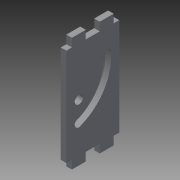
# Autodesk Inventor part: side.plate.cam.rev3
Saved by Autodesk Inventor 2015 SP1 (Build 190203100, 203)
## iProperties
Created: 2016-03-08
Part Number: side.plate.cam.rev3
Material: Generic
Document SubType Name: Modeling
Designer: 200288284
Density: 1 g/cm^3
Appearance: Default
Author: 200288284
Autodesk Inventor part; units mm, degrees
ref_plane "YZ Plane" through (0, 0, 0) normal (1, 0, 0) x (0, 1, 0)
ref_plane "XZ Plane" through (0, 0, 0) normal (0, 1, 0) x (-1, 0, 0)
ref_plane "XY Plane" through (0, 0, 0) normal (0, 0, 1) x (1, 0, 0)
sketch "Sketch1" plane through (0, 0, 0) normal (1, 0, 0) x (0, 1, 0)
  line L0 (8.4448, 10.1682) -> (-26.5552, 10.1682)
  line L1 (-26.5552, 10.1682) -> (-26.5552, 8.1682)
  line L2 (-26.5552, 8.1682) -> (-29.5552, 8.1682)
  line L3 (-29.5552, 8.1682) -> (-29.5552, 3.1682)
  line L4 (-29.5552, 3.1682) -> (-26.5552, 3.1682)
  line L5 (-26.5552, 3.1682) -> (-26.5552, -1.8356)
  line L6 (-26.5552, -1.8356) -> (-29.5552, -1.8356)
  line L7 (-29.5552, -1.8356) -> (-29.5552, -6.8356)
  line L8 (-29.5552, -6.8356) -> (-26.5552, -6.8356)
  line L9 (-26.5552, -6.8356) -> (-26.5552, -8.8356)
  line L10 (-26.5552, -8.8356) -> (8.4448, -8.8356)
  line L11 (11.4448, -1.8356) -> (8.4448, -1.8356)
  line L12 (8.4448, -1.8356) -> (8.4448, 3.1682)
  line L13 (11.4448, 3.1682) -> (8.4448, 3.1682)
  line L14 (11.4448, 3.1682) -> (11.4448, 8.1682)
  line L15 (11.4448, 8.1682) -> (8.4448, 8.1682)
  line L16 (8.4448, 8.1682) -> (8.4448, 10.1682)
  line L17 (11.4448, -1.8356) -> (11.4448, -6.8356)
  line L18 (11.4448, -6.8356) -> (8.4448, -6.8356)
  line L19 (8.4448, -6.8356) -> (8.4448, -8.8356)
  circle A0 centre (-9.0552, 5.6682) radius 1.5
  arc A1 (-14.6939, 5.6682) -> (-17.3326, 4.6918) centre (-16.1939, 5.6682) ccw
  arc A2 (0, -5.8356) -> (-0.3019, -2.8663) centre (0, -4.3356) ccw
  arc A3 (-14.6939, 5.6682) -> (0, -2.8356) centre (-1.5952, 11.3548) ccw
  arc A4 (-17.6939, 5.6682) -> (0, -5.8356) centre (-1.5952, 11.0701) ccw
  point P0 (0, 0)
  dimension "d2" = 2
  dimension "d3" = 3
  dimension "d4" = 5
  dimension "d5" = 5.0038
  dimension "d6" = 5
  dimension "d7" = 2
  dimension "d9" = 3
  dimension "d11" = 3
  dimension "d12" = 3
  constraints: 40 end point, 12 point on circle, 11 perpendicular, 10 point on line, 5 centre point, 3 vertical, 1 horizontal
  measures "d2" distance of L0.end L1.end
  measures "d3" distance of L1.end L2.end
  measures "d4" distance of L2.end L3.end
  measures "d5" distance of L4.end L5.end
  measures "d6" distance of L6.end L7.end
  measures "d7" distance of L8.end L9.end
  measures "d9" diameter of A0
  measures "d11" diameter of A1
  measures "d12" diameter of A2
extrude "Extrusion1" add sketch "Sketch1" along normal blind 2
body "Solid1"
